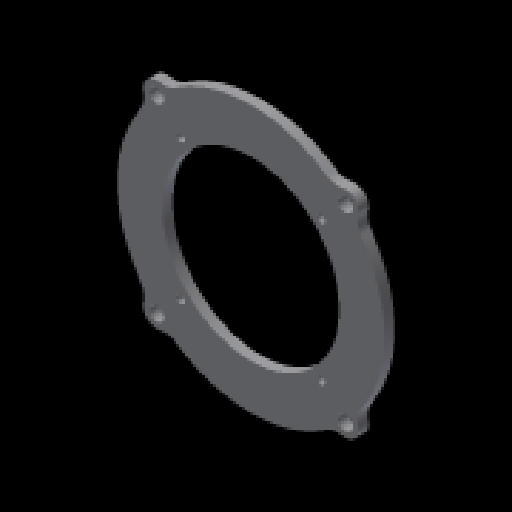
# Autodesk Inventor part: CimCoderMount
Saved by Autodesk Inventor 2025.2 (Build 292293000, 293)
## iProperties
Created: 2026-01-26
Part Number: CimCoderMount
Material: Generic
Document SubType Name: Sheet Metal
Designer: valer
Density: 1 g/cm^3
Appearance: Default
Sheet Metal Rule: Default
Author: valer
Autodesk Inventor part; units mm, degrees
ref_plane "YZ Plane" through (0, 0, 0) normal (1, 0, 0) x (0, 1, 0)
ref_plane "XZ Plane" through (0, 0, 0) normal (0, 1, 0) x (-1, 0, 0)
ref_plane "XY Plane" through (0, 0, 0) normal (0, 0, 1) x (1, 0, 0)
sketch "Base" plane through (0, 0, 0) normal (0, 0, 1) x (1, 0, 0)
  line L0 (-56, 0) -> (56, 0)
  line L1 (0, -56) -> (0, 56) construction
  circle A0 centre (0, 0) radius 40
  line L2 (0, 0) -> (28.2843, 28.2843) construction
  circle A1 centre (28.2843, 28.2843) radius 2.2
  circle A2 centre (-28.2843, 28.2843) radius 2.2
  circle A3 centre (28.2843, -28.2843) radius 2.2
  circle A4 centre (-28.2843, -28.2843) radius 2.2
  circle A5 centre (28.2843, 28.2843) radius 4
  circle A6 centre (-28.2843, 28.2843) radius 4
  circle A7 centre (28.2843, -28.2843) radius 4
  circle A8 centre (-28.2843, -28.2843) radius 4
  circle A9 centre (0, 0) radius 12.2174 construction
  spline S0 degree 3 number of poles 906
  spline S1 degree 3 number of poles 906
  spline S2 degree 3 number of poles 906
  spline S3 degree 3 number of poles 906
  spline S4 degree 2 number of poles 341
  arc A10 (7.6354, -22.3136) -> (7.8387, -21.1617) centre (9.1457, -21.9862) ccw
  circle A11 centre (0, 0) radius 26.5
  point P0 (0, 0)
  point P1 (25.318, 30.9677)
  point P2 (-25.318, 30.9677)
  point P3 (-30.9677, 25.318)
  point P4 (-40, 0)
  point P5 (40, 0)
  point P6 (30.9677, 25.318)
  point P7 (30.9677, -25.318)
  point P8 (-30.9677, -25.318)
  point P9 (-25.318, -30.9677)
  point P10 (25.318, -30.9677)
  point P11 (-29.7965, 26.6864)
  point P12 (-26.6864, 29.7965)
  point P13 (-26.6864, -29.7965)
  point P14 (-29.7965, -26.6864)
extrude "Plate1" add sketch "Base" along normal blind 3 contours A11 L0 A0 A6 A5 | L0 A0 A7 A8 A11 | A5 A0 A1 | A0 A1 A5 | A7 A0 A3 | A0 A3 A7 | A6 A0 A2 | A0 A2 A6 | A8 A0 A4 | A0 A4 A8
fillet "FilletsFeature" radius 6 8 edges at (-30.9677, 25.318, 1.5) (-30.9677, -25.318, 1.5) (-25.318, -30.9677, 1.5) (25.318, -30.9677, 1.5) (30.9677, -25.318, 1.5) (30.9677, 25.318, 1.5) (25.318, 30.9677, 1.5) (-25.318, 30.9677, 1.5)
sketch "WheelEncoderMount" plane through (0, 0, 3) normal (0, 0, 1) x (1, 0, 0)
  circle A0 centre (-20.9919, -21) radius 1.25 projected
  circle A1 centre (-20.9919, 21) radius 1.25 projected
  circle A2 centre (21.0081, -21) radius 1.25 projected
  circle A3 centre (21.0081, 21) radius 1.25 projected
  circle A4 centre (-20.9919, -21) radius 1.25 projected
  circle A5 centre (-20.9919, 21) radius 1.25 projected
  constraints: 4 coincident
hole "EncoderMountHolesFeature" at (-20.9919, -21, 3) at (-20.9919, 21, 3) at (21.0081, 21, 3) at (21.0081, -21, 3) direction (0, 0, -1) diameter 2.45 end through all
equation "\"d48\" = Thickness"
equation "\"d28\" = Thickness"
equation "\"BendRadius\" = Thickness"
equation "\"BendReliefWidth\" = Thickness"
equation "\"BendReliefDepth\" = 0.5 * Thickness"
equation "\"CornerReliefSize\" = 4 * Thickness"
equation "\"MinimumRemnant\" = 2 * Thickness"
equation "\"TransitionRadius\" = BendRadius"
equation "\"JacobiRadiusSize\" = BendRadius"
equation "\"GapSize\" = Thickness"
equation "\"Thickness\" = 3"
body "Solid2"
